Spine Spacer July 13 (Autodesk Fusion 360 design; units mm, degrees)
Autodesk Fusion 360 part; units mm, degrees
sketch "Sketch1" plane through (0, 0, 0) normal (0, 0, 1) x (1, 0, 0)
  line L0 (0, 0) -> (46, 0)
  line L1 (46, 0) -> (46, 20.6)
  line L2 (46, 20.6) -> (0, 20.6)
  line L3 (0, 20.6) -> (0, 0)
  line L4 (0, 20.6) -> (7.7, 20.6)
  line L5 (7.7, 20.6) -> (7.7, 40)
  line L6 (7.7, 40) -> (0, 40)
  line L7 (0, 40) -> (0, 20.6)
  line L8 (7.7, 40) -> (9.4, 40)
  line L9 (9.4, 40) -> (9.4, 32.2)
  line L10 (9.4, 32.2) -> (7.7, 32.2)
  line L11 (7.7, 32.2) -> (7.7, 40)
  line L12 (23, 20.6) -> (23, 0) construction
  line L13 (46, 20.6) -> (38.3, 20.6)
  line L14 (38.3, 20.6) -> (38.3, 40)
  line L15 (46, 40) -> (46, 20.6)
  line L16 (38.3, 40) -> (46, 40)
  line L17 (38.3, 40) -> (36.6, 40)
  line L18 (36.6, 32.2) -> (38.3, 32.2)
  line L19 (38.3, 32.2) -> (38.3, 40)
  line L20 (36.6, 40) -> (36.6, 32.2)
  line L21 (0, 0) -> (-7, 0)
  line L22 (-7, 0) -> (-7, 3)
  line L23 (-7, 3) -> (0, 3)
  line L24 (0, 3) -> (0, 0)
  line L25 (46, 0) -> (53, 0)
  line L26 (53, 0) -> (53, 3)
  line L27 (53, 3) -> (46, 3)
  line L28 (46, 3) -> (46, 0)
  dimension "d1" = 20.6
  dimension "d2" = 46
  dimension "d3" = 7.7
  dimension "d6" = 40
  dimension "d7" = 7.8
  dimension "d8" = 1.7
  dimension "d9" = 7
  dimension "d10" = 3
  dimension "d11" = 3
  dimension "d12" = 7
  measures "d1" distance of L0.start L2.end
  measures "d2" distance of L0.start L0.end
  measures "d3" distance of L5.end L6.end
  measures "d6" distance of L0 L6
  measures "d7" distance of L8.end L9.end
  measures "d8" distance of L5 L9
  measures "d9" distance of L0.start L21.end
  measures "d10" distance of L21.end L22.end
  measures "d11" distance of L25 L27
  measures "d12" distance of L26.end L27.end
extrude "Extrude1" add sketch "Sketch1" along normal blind 20
chamfer "Chamfer1" distance 5 angle 45 1 edges at (23, 0, 20)
sketch "Sketch2" plane through (-7, 0, 0) normal (-1, 0, 0) x (0, 0, 1)
  line L0 (15, 0) -> (18, 3)
  line L1 (18, 3) -> (0, 3)
  line L2 (0, 3) -> (0, 0)
  line L3 (0, 0) -> (15, 0)
  line L4 (5.95, 0) -> (9.05, 0)
  line L5 (9.05, 0) -> (9.05, -1)
  line L6 (9.05, -1) -> (5.95, -1)
  line L7 (5.95, -1) -> (5.95, 0)
  point P0 (7.5, 0)
  dimension "d16" = 1
  dimension "d17" = 3.1
  measures "d16" distance of L4.start L6.end
  measures "d17" distance of L5.end L6.end
extrude "Extrude2" add sketch "Sketch2" against normal up to surface (60 mm away) contours L3 L4 L5 L6 L7
sketch "Sketch3" plane through (0, 0, 0) normal (-1, 0, 0) x (0, 0, 1)
  line L0 (18, 3) -> (20, 5)
  line L1 (20, 5) -> (20, 40)
  line L2 (20, 40) -> (0, 40)
  line L3 (0, 40) -> (0, 3)
  line L4 (0, 3) -> (18, 3)
  circle A0 centre (10, 36.1) radius 3.2
  line L5 (0, 40) -> (0, 32.2)
  point P0 (10, 40)
  point P1 (0, 36.1)
  dimension "d20" = 6.4
  measures "d20" diameter of A0
extrude "Extrude3" cut sketch "Sketch3" against normal through all contours A0
sketch "Sketch4" plane through (0, 40, 0) normal (0, 1, 0) x (-1, 0, 0)
  line L0 (-9.4, 0) -> (0, 0)
  line L1 (0, 0) -> (0, 20)
  line L2 (0, 20) -> (-9.4, 20)
  line L3 (-9.4, 20) -> (-9.4, 0)
  line L4 (0, 0) -> (-7.7, 0)
  line L5 (-7.7, 0) -> (-7.7, 20)
  line L6 (-7.7, 20) -> (0, 20)
  line L7 (0, 20) -> (0, 0)
  point P0 (-7.7, 0)
extrude "Extrude4" add sketch "Sketch4" along normal blind 2 contours L0 L1 L2 L4 L5 L6 L7
ref_plane "WorkPlane1" through (23, 22.5, 10) normal (-1, 0, 0) x (0, -1, 0)
mirror "Mirror1" about plane through (23, 22.5, 10) normal (-1, 0, 0) of "Extrude4"
sketch "Sketch5" plane through (0, 3, 0) normal (0, 1, 0) x (-1, 0, 0)
  line L0 (7, 18) -> (0, 18)
  line L1 (0, 18) -> (0, 0)
  line L2 (0, 0) -> (7, 0)
  line L3 (7, 0) -> (7, 18)
  line L4 (7, 9.05) -> (7, 5.95)
  circle A0 centre (3.5, 7.5) radius 1.75
  point P0 (7, 7.5)
  dimension "d25" = 3.5
  dimension "d26" = 3.5
  measures "d25" diameter of A0
  measures "d26" distance of A0.centre P0
extrude "Extrude5" cut sketch "Sketch5" against normal blind 5 contours A0
mirror "Mirror2" about plane through (23, 22.5, 10) normal (-1, 0, 0) of "Extrude5"
chamfer "Chamfer2" distance 1 angle 45 2 edges at (49.5, 3, 18) (-3.5, 3, 18)
equation "d11 = d10"
equation "d12 = d9"
